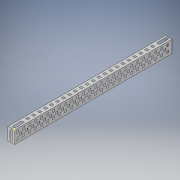
# Autodesk Inventor part: 1sqr x 2sqr metal rail (large)
Saved by Autodesk Inventor 2018 (Build 220112000, 112)
## iProperties
Created: 2018-11-08
Part Number: 1sqr x 2sqr metal rail (large)
Material: Generic
Document SubType Name: Modeling
Designer: USER
Density: 1 g/cm^3
Appearance: Default
Author: USER
Autodesk Inventor part; units mm, degrees
ref_plane "YZ Plane" through (0, 0, 0) normal (1, 0, 0) x (0, 1, 0)
ref_plane "XZ Plane" through (0, 0, 0) normal (0, 1, 0) x (-1, 0, 0)
ref_plane "XY Plane" through (0, 0, 0) normal (0, 0, 1) x (1, 0, 0)
sketch "Sketch1" plane through (0, 0, 0) normal (1, 0, 0) x (0, 1, 0)
  line L0 (0, 0) -> (-25, 0)
  line L1 (-25, 0) -> (-25, -315)
  line L2 (-25, -315) -> (0, -315)
  line L3 (0, -315) -> (0, 0)
  dimension "d0" = 25
  dimension "d1" = 315
  constraints: 8 end point, 2 parallel, 1 horizontal, 1 perpendicular
  measures "d0" distance of L2.end L1.end
  measures "d1" distance of L1.end L0.end
sketch "Sketch2" plane through (0, 0, 0) normal (0, 0, 1) x (1, 0, 0)
  point P0 (0, 0)
sketch "Sketch3" plane through (0, 0, 0) normal (0, 0, 1) x (1, 0, 0)
  line L0 (0, 0) -> (-13, 0)
  line L1 (-13, 0) -> (-13, -25)
  line L2 (-13, -25) -> (0, -25)
  line L3 (0, -25) -> (0, 0)
  dimension "d2" = 13
  dimension "d3" = 25
  constraints: 8 end point, 2 parallel, 1 horizontal, 1 perpendicular
  measures "d2" distance of L2.end L1.end
  measures "d3" distance of L1.end L0.end
sketch "Sketch4" plane through (0, 0, 0) normal (0, 1, 0) x (-1, 0, 0)
  line L0 (0, 0) -> (13, 0)
  line L1 (13, 0) -> (13, -315)
  line L2 (13, -315) -> (0, -315)
  line L3 (0, -315) -> (0, 0)
  dimension "d4" = 13
  dimension "d5" = 315
  constraints: 8 end point, 2 parallel, 1 horizontal, 1 perpendicular
  measures "d4" distance of L1.end L2.end
  measures "d5" distance of L0.end L1.end
sketch "Sketch5" plane through (0, 0, 0) normal (0, 1, 0) x (-1, 0, 0)
  point P0 (0, 0)
sketch "Sketch6" plane through (0, 0, 0) normal (0, 0, 1) x (1, 0, 0)
  point P0 (0, 0)
sketch "Sketch7" plane through (0, 0, 0) normal (0, 0, 1) x (1, 0, 0)
  point P0 (0, 0)
sketch "Sketch8" plane through (0, 0, 0) normal (0, 0, 1) x (1, 0, 0)
  point P0 (0, 0)
extrude "Extrusion1" add sketch "Sketch1" along normal blind 0.1
extrude "Extrusion2" add sketch "Sketch3" along normal blind 0.1 separate body
extrude "Extrusion3" add sketch "Sketch4" along normal blind 0.1 separate body
sketch "Sketch9" plane through (0, 0, -315) normal (0, 0, -1) x (-1, 0, 0)
  line L0 (0, 0) -> (13, 0)
  line L1 (13, 0) -> (13, -25)
  line L2 (13, -25) -> (0, -25)
  line L3 (0, -25) -> (0, 0)
  dimension "d12" = 13
  dimension "d13" = 25
  constraints: 8 end point, 2 parallel, 1 horizontal, 1 perpendicular
  measures "d12" distance of L1.end L2.end
  measures "d13" distance of L0.end L1.end
extrude "Extrusion4" add sketch "Sketch9" along normal blind 0.1 separate body
sketch "Sketch10" plane through (0, 0, -315.1) normal (0, 0, -1) x (-1, 0, 0)
  line L0 (6.3657, -4.7039) -> (6.3657, -20.444) construction
  line L1 (3.8897, -4.7039) -> (3.8897, -20.444)
  line L2 (8.8416, -20.444) -> (8.8416, -4.7039)
  arc A0 (8.8416, -4.7039) -> (3.8897, -4.7039) centre (6.3657, -4.7039) ccw
  arc A1 (3.8897, -20.444) -> (8.8416, -20.444) centre (6.3657, -20.444) ccw
  point P0 (0, 0)
  point P1 (6.3657, -12.574)
  constraints: 8 end point, 4 point on circle, 4 tangent, 2 centre point, 1 midpoint, 1 parallel, 1 vertical
extrude "Extrusion5" cut sketch "Sketch10" against normal blind 508 bodies 4
sketch "Sketch11" plane through (0, 0, 0.1) normal (0, 0, 1) x (1, 0, 0)
  arc A0 (-3.8897, -4.7039) -> (-8.8416, -4.7039) centre (-6.3657, -4.7039) ccw projected
  arc A1 (-8.8416, -20.444) -> (-3.8897, -20.444) centre (-6.3657, -20.444) ccw projected
  line L0 (-6.3657, -4.7039) -> (-6.3657, -20.444) construction
  line L1 (-8.8416, -4.7039) -> (-8.8416, -20.444)
  line L2 (-3.8897, -20.444) -> (-3.8897, -4.7039)
  arc A2 (-3.8897, -4.7039) -> (-8.8416, -4.7039) centre (-6.3657, -4.7039) ccw
  arc A3 (-8.8416, -20.444) -> (-3.8897, -20.444) centre (-6.3657, -20.444) ccw
  point P0 (0, 0)
  point P1 (-6.3657, -12.574)
  constraints: 8 end point, 4 point on circle, 4 tangent, 2 centre point, 1 midpoint, 1 parallel, 1 vertical
extrude "Extrusion6" cut sketch "Sketch11" against normal through all bodies 2
sketch "Sketch12" plane through (0, 0.1, 0) normal (0, 1, 0) x (1, 0, 0)
  line L0 (-6.5, 310.6451) -> (-6.5, 294.8971) construction
  line L1 (-9.3708, 310.6451) -> (-9.3708, 294.8971)
  line L2 (-3.6292, 294.8971) -> (-3.6292, 310.6451)
  arc A0 (-3.6292, 310.6451) -> (-9.3708, 310.6451) centre (-6.5, 310.6451) ccw
  arc A1 (-9.3708, 294.8971) -> (-3.6292, 294.8971) centre (-6.5, 294.8971) ccw
  line L3 (-6.5, 310.6451) -> (9.248, 310.6451) construction
  line L4 (-8.973, 21.463) -> (-8.973, 5.715)
  line L5 (-3.2314, 5.715) -> (-3.2314, 21.463)
  arc A2 (-3.2314, 21.463) -> (-8.973, 21.463) centre (-6.1022, 21.463) ccw
  arc A3 (-8.973, 5.715) -> (-3.2314, 5.715) centre (-6.1022, 5.715) ccw
  line L6 (-4.5149, 285.5533) -> (-9.0869, 285.5533)
  line L7 (-9.0869, 285.5533) -> (-9.0869, 280.9813)
  line L8 (-9.0869, 280.9813) -> (-4.5149, 280.9813)
  line L9 (-4.5149, 280.9813) -> (-4.5149, 285.5533)
  line L10 (-4.5149, 269.0813) -> (-4.5149, 273.6533)
  line L11 (-4.5149, 273.6533) -> (-9.0869, 273.6533)
  line L12 (-9.0869, 273.6533) -> (-9.0869, 269.0813)
  line L13 (-9.0869, 269.0813) -> (-4.5149, 269.0813)
  line L14 (-4.5149, 257.1813) -> (-4.5149, 261.7533)
  line L15 (-4.5149, 261.7533) -> (-9.0869, 261.7533)
  line L16 (-9.0869, 261.7533) -> (-9.0869, 257.1813)
  line L17 (-9.0869, 257.1813) -> (-4.5149, 257.1813)
  line L18 (-4.5149, 245.2813) -> (-4.5149, 249.8533)
  line L19 (-4.5149, 249.8533) -> (-9.0869, 249.8533)
  line L20 (-9.0869, 249.8533) -> (-9.0869, 245.2813)
  line L21 (-9.0869, 245.2813) -> (-4.5149, 245.2813)
  line L22 (-4.5149, 233.3813) -> (-4.5149, 237.9533)
  line L23 (-4.5149, 237.9533) -> (-9.0869, 237.9533)
  line L24 (-9.0869, 237.9533) -> (-9.0869, 233.3813)
  line L25 (-9.0869, 233.3813) -> (-4.5149, 233.3813)
  line L26 (-4.5149, 221.4813) -> (-4.5149, 226.0533)
  line L27 (-4.5149, 226.0533) -> (-9.0869, 226.0533)
  line L28 (-9.0869, 226.0533) -> (-9.0869, 221.4813)
  line L29 (-9.0869, 221.4813) -> (-4.5149, 221.4813)
  line L30 (-4.5149, 209.5813) -> (-4.5149, 214.1533)
  line L31 (-4.5149, 214.1533) -> (-9.0869, 214.1533)
  line L32 (-9.0869, 214.1533) -> (-9.0869, 209.5813)
  line L33 (-9.0869, 209.5813) -> (-4.5149, 209.5813)
  line L34 (-4.5149, 197.6813) -> (-4.5149, 202.2533)
  line L35 (-4.5149, 202.2533) -> (-9.0869, 202.2533)
  line L36 (-9.0869, 202.2533) -> (-9.0869, 197.6813)
  line L37 (-9.0869, 197.6813) -> (-4.5149, 197.6813)
  line L38 (-4.5149, 185.7813) -> (-4.5149, 190.3533)
  line L39 (-4.5149, 190.3533) -> (-9.0869, 190.3533)
  line L40 (-9.0869, 190.3533) -> (-9.0869, 185.7813)
  line L41 (-9.0869, 185.7813) -> (-4.5149, 185.7813)
  line L42 (-4.5149, 173.8813) -> (-4.5149, 178.4533)
  line L43 (-4.5149, 178.4533) -> (-9.0869, 178.4533)
  line L44 (-9.0869, 178.4533) -> (-9.0869, 173.8813)
  line L45 (-9.0869, 173.8813) -> (-4.5149, 173.8813)
  line L46 (-4.5149, 161.9813) -> (-4.5149, 166.5533)
  line L47 (-4.5149, 166.5533) -> (-9.0869, 166.5533)
  line L48 (-9.0869, 166.5533) -> (-9.0869, 161.9813)
  line L49 (-9.0869, 161.9813) -> (-4.5149, 161.9813)
  line L50 (-4.5149, 150.0813) -> (-4.5149, 154.6533)
  line L51 (-4.5149, 154.6533) -> (-9.0869, 154.6533)
  line L52 (-9.0869, 154.6533) -> (-9.0869, 150.0813)
  line L53 (-9.0869, 150.0813) -> (-4.5149, 150.0813)
  line L54 (-4.5149, 138.1813) -> (-4.5149, 142.7533)
  line L55 (-4.5149, 142.7533) -> (-9.0869, 142.7533)
  line L56 (-9.0869, 142.7533) -> (-9.0869, 138.1813)
  line L57 (-9.0869, 138.1813) -> (-4.5149, 138.1813)
  line L58 (-4.5149, 126.2813) -> (-4.5149, 130.8533)
  line L59 (-4.5149, 130.8533) -> (-9.0869, 130.8533)
  line L60 (-9.0869, 130.8533) -> (-9.0869, 126.2813)
  line L61 (-9.0869, 126.2813) -> (-4.5149, 126.2813)
  line L62 (-4.5149, 114.3813) -> (-4.5149, 118.9533)
  line L63 (-4.5149, 118.9533) -> (-9.0869, 118.9533)
  line L64 (-9.0869, 118.9533) -> (-9.0869, 114.3813)
  line L65 (-9.0869, 114.3813) -> (-4.5149, 114.3813)
  line L66 (-4.5149, 102.4813) -> (-4.5149, 107.0533)
  line L67 (-4.5149, 107.0533) -> (-9.0869, 107.0533)
  line L68 (-9.0869, 107.0533) -> (-9.0869, 102.4813)
  line L69 (-9.0869, 102.4813) -> (-4.5149, 102.4813)
  line L70 (-4.5149, 90.5813) -> (-4.5149, 95.1533)
  line L71 (-4.5149, 95.1533) -> (-9.0869, 95.1533)
  line L72 (-9.0869, 95.1533) -> (-9.0869, 90.5813)
  line L73 (-9.0869, 90.5813) -> (-4.5149, 90.5813)
  line L74 (-4.5149, 78.6813) -> (-4.5149, 83.2533)
  line L75 (-4.5149, 83.2533) -> (-9.0869, 83.2533)
  line L76 (-9.0869, 83.2533) -> (-9.0869, 78.6813)
  line L77 (-9.0869, 78.6813) -> (-4.5149, 78.6813)
  line L78 (-4.5149, 66.7813) -> (-4.5149, 71.3533)
  line L79 (-4.5149, 71.3533) -> (-9.0869, 71.3533)
  line L80 (-9.0869, 71.3533) -> (-9.0869, 66.7813)
  line L81 (-9.0869, 66.7813) -> (-4.5149, 66.7813)
  line L82 (-4.5149, 54.8813) -> (-4.5149, 59.4533)
  line L83 (-4.5149, 59.4533) -> (-9.0869, 59.4533)
  line L84 (-9.0869, 59.4533) -> (-9.0869, 54.8813)
  line L85 (-9.0869, 54.8813) -> (-4.5149, 54.8813)
  line L86 (-4.5149, 42.9813) -> (-4.5149, 47.5533)
  line L87 (-4.5149, 47.5533) -> (-9.0869, 47.5533)
  line L88 (-9.0869, 47.5533) -> (-9.0869, 42.9813)
  line L89 (-9.0869, 42.9813) -> (-4.5149, 42.9813)
  line L90 (-4.5149, 31.0813) -> (-4.5149, 35.6533)
  line L91 (-4.5149, 35.6533) -> (-9.0869, 35.6533)
  line L92 (-9.0869, 35.6533) -> (-9.0869, 31.0813)
  line L93 (-9.0869, 31.0813) -> (-4.5149, 31.0813)
  point P0 (0, 0)
  point P1 (-6.5, 302.7711)
  dimension "d20" = 15.748
  dimension "d21" = 90
  dimension "d22" = 15.748
  dimension "d23" = 4.572
  dimension "d24" = 4.572
  dimension "d30" = 11.9
  constraints: 190 end point, 8 point on circle, 8 tangent, 4 centre point, 4 parallel, 2 horizontal, 2 perpendicular, 2 vertical, 1 collinear, 1 midpoint, 167 other
  measures "d20" distance of L0.start L0.end
  measures "d21" angle of L0 L3
  measures "d22" distance of A2.centre A3.centre
  measures "d23" distance of L8.end L7.end
  measures "d24" distance of L7.end L6.end
  measures "d30" distance of L8.end L10.start
extrude "Extrusion7" cut sketch "Sketch12" against normal through all bodies 3
sketch "Sketch13" plane through (0.1, 0, 0) normal (1, 0, 0) x (0, 0, -1)
  line L0 (4.2339, -3.5877) -> (8.8059, -3.5877)
  line L1 (8.8059, -3.5877) -> (8.8059, -8.1597)
  line L2 (8.8059, -8.1597) -> (4.2339, -8.1597)
  line L3 (4.2339, -8.1597) -> (4.2339, -3.5877)
  line L4 (4.2339, -15.5877) -> (8.8059, -15.5877)
  line L5 (4.2339, -20.1597) -> (4.2339, -15.5877)
  line L6 (8.8059, -15.5877) -> (8.8059, -20.1597)
  line L7 (8.8059, -20.1597) -> (4.2339, -20.1597)
  line L8 (16.2339, -3.5877) -> (20.8059, -3.5877)
  line L9 (16.2339, -8.1597) -> (16.2339, -3.5877)
  line L10 (20.8059, -3.5877) -> (20.8059, -8.1597)
  line L11 (20.8059, -8.1597) -> (16.2339, -8.1597)
  line L12 (16.2339, -15.5877) -> (20.8059, -15.5877)
  line L13 (16.2339, -20.1597) -> (16.2339, -15.5877)
  line L14 (20.8059, -15.5877) -> (20.8059, -20.1597)
  line L15 (20.8059, -20.1597) -> (16.2339, -20.1597)
  line L16 (28.2339, -3.5877) -> (32.8059, -3.5877)
  line L17 (28.2339, -8.1597) -> (28.2339, -3.5877)
  line L18 (32.8059, -3.5877) -> (32.8059, -8.1597)
  line L19 (32.8059, -8.1597) -> (28.2339, -8.1597)
  line L20 (28.2339, -15.5877) -> (32.8059, -15.5877)
  line L21 (28.2339, -20.1597) -> (28.2339, -15.5877)
  line L22 (32.8059, -15.5877) -> (32.8059, -20.1597)
  line L23 (32.8059, -20.1597) -> (28.2339, -20.1597)
  line L24 (40.2339, -3.5877) -> (44.8059, -3.5877)
  line L25 (40.2339, -8.1597) -> (40.2339, -3.5877)
  line L26 (44.8059, -3.5877) -> (44.8059, -8.1597)
  line L27 (44.8059, -8.1597) -> (40.2339, -8.1597)
  line L28 (40.2339, -15.5877) -> (44.8059, -15.5877)
  line L29 (40.2339, -20.1597) -> (40.2339, -15.5877)
  line L30 (44.8059, -15.5877) -> (44.8059, -20.1597)
  line L31 (44.8059, -20.1597) -> (40.2339, -20.1597)
  line L32 (52.2339, -3.5877) -> (56.8059, -3.5877)
  line L33 (52.2339, -8.1597) -> (52.2339, -3.5877)
  line L34 (56.8059, -3.5877) -> (56.8059, -8.1597)
  line L35 (56.8059, -8.1597) -> (52.2339, -8.1597)
  line L36 (52.2339, -15.5877) -> (56.8059, -15.5877)
  line L37 (52.2339, -20.1597) -> (52.2339, -15.5877)
  line L38 (56.8059, -15.5877) -> (56.8059, -20.1597)
  line L39 (56.8059, -20.1597) -> (52.2339, -20.1597)
  line L40 (64.2339, -3.5877) -> (68.8059, -3.5877)
  line L41 (64.2339, -8.1597) -> (64.2339, -3.5877)
  line L42 (68.8059, -3.5877) -> (68.8059, -8.1597)
  line L43 (68.8059, -8.1597) -> (64.2339, -8.1597)
  line L44 (64.2339, -15.5877) -> (68.8059, -15.5877)
  line L45 (64.2339, -20.1597) -> (64.2339, -15.5877)
  line L46 (68.8059, -15.5877) -> (68.8059, -20.1597)
  line L47 (68.8059, -20.1597) -> (64.2339, -20.1597)
  line L48 (76.2339, -3.5877) -> (80.8059, -3.5877)
  line L49 (76.2339, -8.1597) -> (76.2339, -3.5877)
  line L50 (80.8059, -3.5877) -> (80.8059, -8.1597)
  line L51 (80.8059, -8.1597) -> (76.2339, -8.1597)
  line L52 (76.2339, -15.5877) -> (80.8059, -15.5877)
  line L53 (76.2339, -20.1597) -> (76.2339, -15.5877)
  line L54 (80.8059, -15.5877) -> (80.8059, -20.1597)
  line L55 (80.8059, -20.1597) -> (76.2339, -20.1597)
  line L56 (88.2339, -3.5877) -> (92.8059, -3.5877)
  line L57 (88.2339, -8.1597) -> (88.2339, -3.5877)
  line L58 (92.8059, -3.5877) -> (92.8059, -8.1597)
  line L59 (92.8059, -8.1597) -> (88.2339, -8.1597)
  line L60 (88.2339, -15.5877) -> (92.8059, -15.5877)
  line L61 (88.2339, -20.1597) -> (88.2339, -15.5877)
  line L62 (92.8059, -15.5877) -> (92.8059, -20.1597)
  line L63 (92.8059, -20.1597) -> (88.2339, -20.1597)
  line L64 (100.2339, -3.5877) -> (104.8059, -3.5877)
  line L65 (100.2339, -8.1597) -> (100.2339, -3.5877)
  line L66 (104.8059, -3.5877) -> (104.8059, -8.1597)
  line L67 (104.8059, -8.1597) -> (100.2339, -8.1597)
  line L68 (100.2339, -15.5877) -> (104.8059, -15.5877)
  line L69 (100.2339, -20.1597) -> (100.2339, -15.5877)
  line L70 (104.8059, -15.5877) -> (104.8059, -20.1597)
  line L71 (104.8059, -20.1597) -> (100.2339, -20.1597)
  line L72 (112.2339, -3.5877) -> (116.8059, -3.5877)
  line L73 (112.2339, -8.1597) -> (112.2339, -3.5877)
  line L74 (116.8059, -3.5877) -> (116.8059, -8.1597)
  line L75 (116.8059, -8.1597) -> (112.2339, -8.1597)
  line L76 (112.2339, -15.5877) -> (116.8059, -15.5877)
  line L77 (112.2339, -20.1597) -> (112.2339, -15.5877)
  line L78 (116.8059, -15.5877) -> (116.8059, -20.1597)
  line L79 (116.8059, -20.1597) -> (112.2339, -20.1597)
  line L80 (124.2339, -3.5877) -> (128.8059, -3.5877)
  line L81 (124.2339, -8.1597) -> (124.2339, -3.5877)
  line L82 (128.8059, -3.5877) -> (128.8059, -8.1597)
  line L83 (128.8059, -8.1597) -> (124.2339, -8.1597)
  line L84 (124.2339, -15.5877) -> (128.8059, -15.5877)
  line L85 (124.2339, -20.1597) -> (124.2339, -15.5877)
  line L86 (128.8059, -15.5877) -> (128.8059, -20.1597)
  line L87 (128.8059, -20.1597) -> (124.2339, -20.1597)
  line L88 (136.2339, -3.5877) -> (140.8059, -3.5877)
  line L89 (136.2339, -8.1597) -> (136.2339, -3.5877)
  line L90 (140.8059, -3.5877) -> (140.8059, -8.1597)
  line L91 (140.8059, -8.1597) -> (136.2339, -8.1597)
  line L92 (136.2339, -15.5877) -> (140.8059, -15.5877)
  line L93 (136.2339, -20.1597) -> (136.2339, -15.5877)
  line L94 (140.8059, -15.5877) -> (140.8059, -20.1597)
  line L95 (140.8059, -20.1597) -> (136.2339, -20.1597)
  line L96 (148.2339, -3.5877) -> (152.8059, -3.5877)
  line L97 (148.2339, -8.1597) -> (148.2339, -3.5877)
  line L98 (152.8059, -3.5877) -> (152.8059, -8.1597)
  line L99 (152.8059, -8.1597) -> (148.2339, -8.1597)
  line L100 (148.2339, -15.5877) -> (152.8059, -15.5877)
  line L101 (148.2339, -20.1597) -> (148.2339, -15.5877)
  line L102 (152.8059, -15.5877) -> (152.8059, -20.1597)
  line L103 (152.8059, -20.1597) -> (148.2339, -20.1597)
  line L104 (160.2339, -3.5877) -> (164.8059, -3.5877)
  line L105 (160.2339, -8.1597) -> (160.2339, -3.5877)
  line L106 (164.8059, -3.5877) -> (164.8059, -8.1597)
  line L107 (164.8059, -8.1597) -> (160.2339, -8.1597)
  line L108 (160.2339, -15.5877) -> (164.8059, -15.5877)
  line L109 (160.2339, -20.1597) -> (160.2339, -15.5877)
  line L110 (164.8059, -15.5877) -> (164.8059, -20.1597)
  line L111 (164.8059, -20.1597) -> (160.2339, -20.1597)
  line L112 (172.2339, -3.5877) -> (176.8059, -3.5877)
  line L113 (172.2339, -8.1597) -> (172.2339, -3.5877)
  line L114 (176.8059, -3.5877) -> (176.8059, -8.1597)
  line L115 (176.8059, -8.1597) -> (172.2339, -8.1597)
  line L116 (172.2339, -15.5877) -> (176.8059, -15.5877)
  line L117 (172.2339, -20.1597) -> (172.2339, -15.5877)
  line L118 (176.8059, -15.5877) -> (176.8059, -20.1597)
  line L119 (176.8059, -20.1597) -> (172.2339, -20.1597)
  line L120 (184.2339, -3.5877) -> (188.8059, -3.5877)
  line L121 (184.2339, -8.1597) -> (184.2339, -3.5877)
  line L122 (188.8059, -3.5877) -> (188.8059, -8.1597)
  line L123 (188.8059, -8.1597) -> (184.2339, -8.1597)
  line L124 (184.2339, -15.5877) -> (188.8059, -15.5877)
  line L125 (184.2339, -20.1597) -> (184.2339, -15.5877)
  line L126 (188.8059, -15.5877) -> (188.8059, -20.1597)
  line L127 (188.8059, -20.1597) -> (184.2339, -20.1597)
  line L128 (196.2339, -3.5877) -> (200.8059, -3.5877)
  line L129 (196.2339, -8.1597) -> (196.2339, -3.5877)
  line L130 (200.8059, -3.5877) -> (200.8059, -8.1597)
  line L131 (200.8059, -8.1597) -> (196.2339, -8.1597)
  line L132 (196.2339, -15.5877) -> (200.8059, -15.5877)
  line L133 (196.2339, -20.1597) -> (196.2339, -15.5877)
  line L134 (200.8059, -15.5877) -> (200.8059, -20.1597)
  line L135 (200.8059, -20.1597) -> (196.2339, -20.1597)
  line L136 (208.2339, -3.5877) -> (212.8059, -3.5877)
  line L137 (208.2339, -8.1597) -> (208.2339, -3.5877)
  line L138 (212.8059, -3.5877) -> (212.8059, -8.1597)
  line L139 (212.8059, -8.1597) -> (208.2339, -8.1597)
  line L140 (208.2339, -15.5877) -> (212.8059, -15.5877)
  line L141 (208.2339, -20.1597) -> (208.2339, -15.5877)
  line L142 (212.8059, -15.5877) -> (212.8059, -20.1597)
  line L143 (212.8059, -20.1597) -> (208.2339, -20.1597)
  line L144 (220.2339, -3.5877) -> (224.8059, -3.5877)
  line L145 (220.2339, -8.1597) -> (220.2339, -3.5877)
  line L146 (224.8059, -3.5877) -> (224.8059, -8.1597)
  line L147 (224.8059, -8.1597) -> (220.2339, -8.1597)
  line L148 (220.2339, -15.5877) -> (224.8059, -15.5877)
  line L149 (220.2339, -20.1597) -> (220.2339, -15.5877)
  line L150 (224.8059, -15.5877) -> (224.8059, -20.1597)
  line L151 (224.8059, -20.1597) -> (220.2339, -20.1597)
  line L152 (232.2339, -3.5877) -> (236.8059, -3.5877)
  line L153 (232.2339, -8.1597) -> (232.2339, -3.5877)
  line L154 (236.8059, -3.5877) -> (236.8059, -8.1597)
  line L155 (236.8059, -8.1597) -> (232.2339, -8.1597)
  line L156 (232.2339, -15.5877) -> (236.8059, -15.5877)
  line L157 (232.2339, -20.1597) -> (232.2339, -15.5877)
  line L158 (236.8059, -15.5877) -> (236.8059, -20.1597)
  line L159 (236.8059, -20.1597) -> (232.2339, -20.1597)
  line L160 (244.2339, -3.5877) -> (248.8059, -3.5877)
  line L161 (244.2339, -8.1597) -> (244.2339, -3.5877)
  line L162 (248.8059, -3.5877) -> (248.8059, -8.1597)
  line L163 (248.8059, -8.1597) -> (244.2339, -8.1597)
  line L164 (244.2339, -15.5877) -> (248.8059, -15.5877)
  line L165 (244.2339, -20.1597) -> (244.2339, -15.5877)
  line L166 (248.8059, -15.5877) -> (248.8059, -20.1597)
  line L167 (248.8059, -20.1597) -> (244.2339, -20.1597)
  line L168 (256.2339, -3.5877) -> (260.8059, -3.5877)
  line L169 (256.2339, -8.1597) -> (256.2339, -3.5877)
  line L170 (260.8059, -3.5877) -> (260.8059, -8.1597)
  line L171 (260.8059, -8.1597) -> (256.2339, -8.1597)
  line L172 (256.2339, -15.5877) -> (260.8059, -15.5877)
  line L173 (256.2339, -20.1597) -> (256.2339, -15.5877)
  line L174 (260.8059, -15.5877) -> (260.8059, -20.1597)
  line L175 (260.8059, -20.1597) -> (256.2339, -20.1597)
  line L176 (268.2339, -3.5877) -> (272.8059, -3.5877)
  line L177 (268.2339, -8.1597) -> (268.2339, -3.5877)
  line L178 (272.8059, -3.5877) -> (272.8059, -8.1597)
  line L179 (272.8059, -8.1597) -> (268.2339, -8.1597)
  line L180 (268.2339, -15.5877) -> (272.8059, -15.5877)
  line L181 (268.2339, -20.1597) -> (268.2339, -15.5877)
  line L182 (272.8059, -15.5877) -> (272.8059, -20.1597)
  line L183 (272.8059, -20.1597) -> (268.2339, -20.1597)
  line L184 (280.2339, -3.5877) -> (284.8059, -3.5877)
  line L185 (280.2339, -8.1597) -> (280.2339, -3.5877)
  line L186 (284.8059, -3.5877) -> (284.8059, -8.1597)
  line L187 (284.8059, -8.1597) -> (280.2339, -8.1597)
  line L188 (280.2339, -15.5877) -> (284.8059, -15.5877)
  line L189 (280.2339, -20.1597) -> (280.2339, -15.5877)
  line L190 (284.8059, -15.5877) -> (284.8059, -20.1597)
  line L191 (284.8059, -20.1597) -> (280.2339, -20.1597)
  line L192 (292.2339, -3.5877) -> (296.8059, -3.5877)
  line L193 (292.2339, -8.1597) -> (292.2339, -3.5877)
  line L194 (296.8059, -3.5877) -> (296.8059, -8.1597)
  line L195 (296.8059, -8.1597) -> (292.2339, -8.1597)
  line L196 (292.2339, -15.5877) -> (296.8059, -15.5877)
  line L197 (292.2339, -20.1597) -> (292.2339, -15.5877)
  line L198 (296.8059, -15.5877) -> (296.8059, -20.1597)
  line L199 (296.8059, -20.1597) -> (292.2339, -20.1597)
  line L200 (304.2339, -3.5877) -> (308.8059, -3.5877)
  line L201 (304.2339, -8.1597) -> (304.2339, -3.5877)
  line L202 (308.8059, -3.5877) -> (308.8059, -8.1597)
  line L203 (308.8059, -8.1597) -> (304.2339, -8.1597)
  line L204 (304.2339, -15.5877) -> (308.8059, -15.5877)
  line L205 (304.2339, -20.1597) -> (304.2339, -15.5877)
  line L206 (308.8059, -15.5877) -> (308.8059, -20.1597)
  line L207 (308.8059, -20.1597) -> (304.2339, -20.1597)
  line L208 (9.8139, -9.5549) -> (14.3859, -9.5549)
  line L209 (14.3859, -9.5549) -> (14.3859, -14.1269)
  line L210 (14.3859, -14.1269) -> (9.8139, -14.1269)
  line L211 (9.8139, -14.1269) -> (9.8139, -9.5549)
  line L212 (21.8139, -9.5549) -> (26.3859, -9.5549)
  line L213 (21.8139, -14.1269) -> (21.8139, -9.5549)
  line L214 (26.3859, -14.1269) -> (21.8139, -14.1269)
  line L215 (26.3859, -9.5549) -> (26.3859, -14.1269)
  line L216 (33.8139, -9.5549) -> (38.3859, -9.5549)
  line L217 (33.8139, -14.1269) -> (33.8139, -9.5549)
  line L218 (38.3859, -14.1269) -> (33.8139, -14.1269)
  line L219 (38.3859, -9.5549) -> (38.3859, -14.1269)
  line L220 (45.8139, -9.5549) -> (50.3859, -9.5549)
  line L221 (45.8139, -14.1269) -> (45.8139, -9.5549)
  line L222 (50.3859, -14.1269) -> (45.8139, -14.1269)
  line L223 (50.3859, -9.5549) -> (50.3859, -14.1269)
  line L224 (57.8139, -9.5549) -> (62.3859, -9.5549)
  line L225 (57.8139, -14.1269) -> (57.8139, -9.5549)
  line L226 (62.3859, -14.1269) -> (57.8139, -14.1269)
  line L227 (62.3859, -9.5549) -> (62.3859, -14.1269)
  line L228 (69.8139, -9.5549) -> (74.3859, -9.5549)
  line L229 (69.8139, -14.1269) -> (69.8139, -9.5549)
  line L230 (74.3859, -14.1269) -> (69.8139, -14.1269)
  line L231 (74.3859, -9.5549) -> (74.3859, -14.1269)
  line L232 (81.8139, -9.5549) -> (86.3859, -9.5549)
  line L233 (81.8139, -14.1269) -> (81.8139, -9.5549)
  line L234 (86.3859, -14.1269) -> (81.8139, -14.1269)
  line L235 (86.3859, -9.5549) -> (86.3859, -14.1269)
  line L236 (93.8139, -9.5549) -> (98.3859, -9.5549)
  line L237 (93.8139, -14.1269) -> (93.8139, -9.5549)
  line L238 (98.3859, -14.1269) -> (93.8139, -14.1269)
  line L239 (98.3859, -9.5549) -> (98.3859, -14.1269)
  line L240 (105.8139, -9.5549) -> (110.3859, -9.5549)
  line L241 (105.8139, -14.1269) -> (105.8139, -9.5549)
  line L242 (110.3859, -14.1269) -> (105.8139, -14.1269)
  line L243 (110.3859, -9.5549) -> (110.3859, -14.1269)
  line L244 (117.8139, -9.5549) -> (122.3859, -9.5549)
  line L245 (117.8139, -14.1269) -> (117.8139, -9.5549)
  line L246 (122.3859, -14.1269) -> (117.8139, -14.1269)
  line L247 (122.3859, -9.5549) -> (122.3859, -14.1269)
  line L248 (129.8139, -9.5549) -> (134.3859, -9.5549)
  line L249 (129.8139, -14.1269) -> (129.8139, -9.5549)
  line L250 (134.3859, -14.1269) -> (129.8139, -14.1269)
  line L251 (134.3859, -9.5549) -> (134.3859, -14.1269)
  line L252 (141.8139, -9.5549) -> (146.3859, -9.5549)
  line L253 (141.8139, -14.1269) -> (141.8139, -9.5549)
  line L254 (146.3859, -14.1269) -> (141.8139, -14.1269)
  line L255 (146.3859, -9.5549) -> (146.3859, -14.1269)
  line L256 (153.8139, -9.5549) -> (158.3859, -9.5549)
  line L257 (153.8139, -14.1269) -> (153.8139, -9.5549)
  line L258 (158.3859, -14.1269) -> (153.8139, -14.1269)
  line L259 (158.3859, -9.5549) -> (158.3859, -14.1269)
  line L260 (165.8139, -9.5549) -> (170.3859, -9.5549)
  line L261 (165.8139, -14.1269) -> (165.8139, -9.5549)
  line L262 (170.3859, -14.1269) -> (165.8139, -14.1269)
  line L263 (170.3859, -9.5549) -> (170.3859, -14.1269)
  line L264 (177.8139, -9.5549) -> (182.3859, -9.5549)
  line L265 (177.8139, -14.1269) -> (177.8139, -9.5549)
  line L266 (182.3859, -14.1269) -> (177.8139, -14.1269)
  line L267 (182.3859, -9.5549) -> (182.3859, -14.1269)
  line L268 (189.8139, -9.5549) -> (194.3859, -9.5549)
  line L269 (189.8139, -14.1269) -> (189.8139, -9.5549)
  line L270 (194.3859, -14.1269) -> (189.8139, -14.1269)
  line L271 (194.3859, -9.5549) -> (194.3859, -14.1269)
  line L272 (201.8139, -9.5549) -> (206.3859, -9.5549)
  line L273 (201.8139, -14.1269) -> (201.8139, -9.5549)
  line L274 (206.3859, -14.1269) -> (201.8139, -14.1269)
  line L275 (206.3859, -9.5549) -> (206.3859, -14.1269)
  line L276 (213.8139, -9.5549) -> (218.3859, -9.5549)
  line L277 (213.8139, -14.1269) -> (213.8139, -9.5549)
  line L278 (218.3859, -14.1269) -> (213.8139, -14.1269)
  line L279 (218.3859, -9.5549) -> (218.3859, -14.1269)
  line L280 (225.8139, -9.5549) -> (230.3859, -9.5549)
  line L281 (225.8139, -14.1269) -> (225.8139, -9.5549)
  line L282 (230.3859, -14.1269) -> (225.8139, -14.1269)
  line L283 (230.3859, -9.5549) -> (230.3859, -14.1269)
  line L284 (237.8139, -9.5549) -> (242.3859, -9.5549)
  line L285 (237.8139, -14.1269) -> (237.8139, -9.5549)
  line L286 (242.3859, -14.1269) -> (237.8139, -14.1269)
  line L287 (242.3859, -9.5549) -> (242.3859, -14.1269)
  line L288 (249.8139, -9.5549) -> (254.3859, -9.5549)
  line L289 (249.8139, -14.1269) -> (249.8139, -9.5549)
  line L290 (254.3859, -14.1269) -> (249.8139, -14.1269)
  line L291 (254.3859, -9.5549) -> (254.3859, -14.1269)
  line L292 (261.8139, -9.5549) -> (266.3859, -9.5549)
  line L293 (261.8139, -14.1269) -> (261.8139, -9.5549)
  line L294 (266.3859, -14.1269) -> (261.8139, -14.1269)
  line L295 (266.3859, -9.5549) -> (266.3859, -14.1269)
  line L296 (273.8139, -9.5549) -> (278.3859, -9.5549)
  line L297 (273.8139, -14.1269) -> (273.8139, -9.5549)
  line L298 (278.3859, -14.1269) -> (273.8139, -14.1269)
  line L299 (278.3859, -9.5549) -> (278.3859, -14.1269)
  line L300 (285.8139, -9.5549) -> (290.3859, -9.5549)
  line L301 (285.8139, -14.1269) -> (285.8139, -9.5549)
  line L302 (290.3859, -14.1269) -> (285.8139, -14.1269)
  line L303 (290.3859, -9.5549) -> (290.3859, -14.1269)
  line L304 (297.8139, -9.5549) -> (302.3859, -9.5549)
  line L305 (297.8139, -14.1269) -> (297.8139, -9.5549)
  line L306 (302.3859, -14.1269) -> (297.8139, -14.1269)
  line L307 (302.3859, -9.5549) -> (302.3859, -14.1269)
  point P0 (0, 0)
  dimension "d34" = 4.572
  dimension "d35" = 4.572
  dimension "d38" = 12
  dimension "d41" = 12
  dimension "d44" = 4.572
  dimension "d45" = 4.572
  dimension "d51" = 12
  constraints: 616 end point, 4 horizontal, 4 parallel, 3 collinear, 2 perpendicular, 1 vertical, 597 other
  measures "d34" distance of L1.end L2.end
  measures "d35" distance of L0.end L1.end
  measures "d38" distance of L0.start L4.start
  measures "d41" distance of L0.start L8.start
  measures "d44" distance of L209.end L210.end
  measures "d45" distance of L208.end L209.end
  measures "d51" distance of L208.start L212.start
extrude "Extrusion8" cut sketch "Sketch13" against normal through all bodies 1
body "Solid1"
body "Solid2"
body "Solid3"
body "Solid4"
